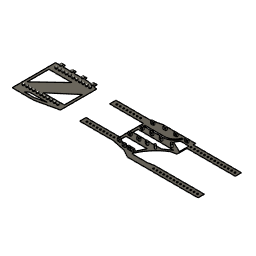
palm&backhand v9 (Autodesk Fusion 360 design; units mm, degrees)
Autodesk Fusion 360 part; units mm, degrees
(part 1 of 4)
sketch "Sketch1" plane through (0, 0, 0) normal (0, 0, 1) x (1, 0, 0)
  line L0 (90, 80) -> (90, -10)
  line L1 (45, 80) -> (45, -10) construction
  line L2 (45, -10) -> (0, 0)
  line L3 (45, -10) -> (90, -10)
  line L4 (22.5, 80) -> (90, 80)
  line L5 (22.5, 80) -> (0, 75)
  line L6 (0, 0) -> (0, 75)
  line L7 (90, 80) -> (90, 40) construction
  arc A0 (90, 40) -> (45, -10) centre (128.4491, -39.8542) ccw
  arc A1 (87.8309, 44.505) -> (40.2922, -8.3158) centre (128.4491, -39.8542) ccw
  line L8 (87.8309, 44.505) -> (87.8309, 38.9188)
  line L9 (87.8309, 44.505) -> (90, 44.58)
  line L10 (40.6089, -7.444) -> (45.6219, -8.3158)
  line L11 (40.2922, -8.3158) -> (40.0807, -8.9068)
  line L12 (0, 0) -> (-30, 0)
  line L13 (-30, 0) -> (-30, 75)
  line L14 (-30, 75) -> (0, 75)
  line L15 (-30, 5) -> (0, 5)
  line L16 (-30, 70) -> (0, 70)
  line L17 (-75, -10) -> (-30, 0)
  line L18 (-117.8309, 44.505) -> (-117.8309, 38.9188)
  line L19 (-70.6089, -7.444) -> (-75.6219, -8.3158)
  line L20 (-120, 80) -> (-120, 40) construction
  line L21 (-120, 80) -> (-120, -10)
  line L22 (-75, 80) -> (-75, -10) construction
  arc A2 (-120, 40) -> (-75, -10) centre (-158.4491, -39.8542) cw
  line L23 (-52.5, 80) -> (-120, 80)
  arc A3 (-117.8309, 44.505) -> (-70.2922, -8.3158) centre (-158.4491, -39.8542) cw
  line L24 (-70.2922, -8.3158) -> (-70.0807, -8.9068)
  line L25 (-117.8309, 44.505) -> (-120, 44.58)
  line L26 (-75, -10) -> (-120, -10)
  line L27 (-52.5, 80) -> (-30, 75)
  line L28 (90, 80) -> (90, 75)
  line L29 (90, 44.58) -> (89.8272, 49.577)
  line L30 (90, 75) -> (190, 75)
  line L31 (75.7574, -10) -> (181.8234, -116.066)
  line L32 (181.8234, -116.066) -> (195.9655, -101.9239)
  line L33 (195.9655, -101.9239) -> (89.8995, 4.1421)
  line L34 (89.8995, 4.1421) -> (75.7574, -10)
  circle A4 centre (187.1267, -107.2272) radius 2.5 construction
  circle A5 centre (181.8234, -101.9239) radius 5
  circle A6 centre (174.7523, -94.8528) radius 5 construction
  circle A7 centre (167.6812, -87.7817) radius 5
  circle A8 centre (160.6102, -80.7107) radius 5 construction
  circle A9 centre (153.5391, -73.6396) radius 5
  circle A10 centre (146.468, -66.5685) radius 5 construction
  circle A11 centre (139.397, -59.4975) radius 5
  circle A12 centre (132.3259, -52.4264) radius 5 construction
  line L35 (188.8944, -108.9949) -> (82.8284, -2.9289) construction
  circle A13 centre (125.2548, -45.3553) radius 5
  circle A14 centre (118.1838, -38.2843) radius 5 construction
  circle A15 centre (111.1127, -31.2132) radius 5
  line L36 (190, 62.2885) -> (90, 62.2885)
  line L37 (90, 75) -> (90, 62.2885)
  line L38 (190, 62.2885) -> (190, 75)
  line L39 (190, 68.6442) -> (90, 68.6442) construction
  circle A16 centre (187.5, 68.6442) radius 2.5 construction
  circle A17 centre (180, 68.6442) radius 5
  circle A18 centre (170, 68.6442) radius 5 construction
  circle A19 centre (160, 68.6442) radius 5
  circle A20 centre (150, 68.6442) radius 5 construction
  circle A21 centre (140, 68.6442) radius 5
  circle A22 centre (130, 68.6442) radius 5 construction
  circle A23 centre (120, 68.6442) radius 5
  circle A24 centre (111.1127, -31.2132) radius 4.5
  circle A25 centre (125.2548, -45.3553) radius 4.5
  circle A26 centre (139.397, -59.4975) radius 4.5
  circle A27 centre (153.5391, -73.6396) radius 4.5
  circle A28 centre (167.6812, -87.7817) radius 4.5
  circle A29 centre (181.8234, -101.9239) radius 4.5
  circle A30 centre (104.0416, -24.1421) radius 5 construction
  circle A31 centre (96.9706, -17.0711) radius 5 construction
  circle A32 centre (96.9706, -17.0711) radius 4.5
  dimension "d3" = 90
  dimension "d4" = 90
  dimension "d7" = 40
  dimension "d8" = 5
  dimension "d9" = 30
  dimension "d13" = 90
  dimension "d14" = 90
  dimension "d15" = 40
  dimension "d16" = 5
  dimension "d17" = 5
  dimension "d18" = 100
  dimension "d20" = 150
  dimension "d22" = 5
  dimension "d23" = 10
  dimension "d24" = 10
  dimension "d25" = 10
  dimension "d26" = 10
  dimension "d27" = 10
  dimension "d28" = 10
  dimension "d29" = 10
  dimension "d30" = 10
  dimension "d31" = 10
  dimension "d32" = 10
  dimension "d33" = 10
  dimension "d34" = 5
  dimension "d35" = 10
  dimension "d36" = 10
  dimension "d37" = 10
  dimension "d38" = 10
  dimension "d39" = 10
  dimension "d40" = 10
  dimension "d41" = 10
  dimension "d465" = 9
  dimension "d466" = 9
  dimension "d467" = 9
  dimension "d468" = 9
  dimension "d469" = 9
  dimension "d470" = 9
  dimension "d539" = 10
  dimension "d540" = 10
  dimension "d541" = 9
  constraint coincident L2.end L6.start
  constraint perpendicular L0 L4
  constraint vertical L6
  constraint perpendicular L4 L7
  constraint coincident A0 L8.end
  constraint vertical L8
  constraint coincident L0 L9.end
  constraint coincident A1 L10.start
  constraint coincident A0 L10.end
  constraint coincident L2 L11.end
  constraint tangent A1 L11
  constraint perpendicular L6 L12
  constraint perpendicular L12 L13
  constraint perpendicular L6 L14
  constraint coincident L13 L15.start
  constraint coincident L6 L15.end
  constraint perpendicular L6 L15
  constraint coincident L13 L16.start
  constraint coincident L6 L16.end
  constraint perpendicular L6 L16
  constraint perpendicular L21 L23
  constraint perpendicular L20 L23
  constraint coincident L18.end A2
  constraint coincident L25.end L21
  constraint coincident L19.start A3
  constraint coincident L19.end A2
  constraint coincident L24.end L17
  constraint tangent A3 L24
  constraint concentric A2 A3
  constraint perpendicular L4 L28
  constraint perpendicular L9 L29
  constraint horizontal L30
  constraint midpoint L32 L35.start
  constraint midpoint L34 L35.end
  constraint perpendicular L0 L36
  constraint perpendicular L36 L37
  constraint perpendicular L30 L38
  constraint midpoint L38 L39.start
  constraint midpoint L37 L39.end
  constraint perpendicular L7 L39
  constraint coincident L39.start A16
  constraint concentric A15 A24
  constraint concentric A13 A25
  constraint concentric A11 A26
  constraint concentric A9 A27
  constraint concentric A7 A28
  constraint concentric A5 A29
  constraint concentric A31 A32
  measures "d3" distance of L0.start L0.end
  measures "d4" distance of L1.start L1.end
  measures "d7" distance of L0.start L7.end
  measures "d9" distance of L2.end L12.end
  measures "d13" distance of L21.end L20.start
  measures "d14" distance of L17.start L22.start
  measures "d15" distance of L20.end L20.start
  measures "d16" distance of L0.start L28.end
  measures "d17" distance of L9.end L29.end
  measures "d18" distance of L28.end L30.end
  measures "d20" distance of L31.start L31.end
  measures "d22" diameter of A4
  measures "d23" diameter of A5
  measures "d24" diameter of A6
  measures "d25" diameter of A7
  measures "d26" diameter of A8
  measures "d27" diameter of A9
  measures "d28" diameter of A10
  measures "d29" diameter of A11
  measures "d30" diameter of A12
  measures "d31" diameter of A13
  measures "d32" diameter of A14
  measures "d33" diameter of A15
  measures "d34" diameter of A16
  measures "d35" diameter of A17
  measures "d36" diameter of A18
  measures "d37" diameter of A19
  measures "d38" diameter of A20
  measures "d39" diameter of A21
  measures "d40" diameter of A22
  measures "d41" diameter of A23
  measures "d465" diameter of A24
  measures "d466" diameter of A25
  measures "d467" diameter of A26
  measures "d468" diameter of A27
  measures "d469" diameter of A28
  measures "d470" diameter of A29
  measures "d539" diameter of A30
  measures "d540" diameter of A31
  measures "d541" diameter of A32
extrude "Extrude1" add sketch "Sketch1" along normal blind 0.5 contours L0 L2 L4 L5 L6 A1 L9 L11 L28 L37 | L0 L30 L36 L37 L38 | L6 L13 L14 L16 | L0 A0 L8 L9 | L13 L17 L21 L23 A3 L24 L25 L27 | L0 L3 A0 L33 L34 | L6 L12 L13 L15 | L0 L3 L31 L32 L33 | L0 L3 L33 L34 | L2 A0 A1 L10 L11 | L18 L21 A2 L25 | L17 L19 A2 A3 L24 | L21 A2 L26 | L18 L19 A2 A3 | A32 makes body 1
sketch "Sketch2" plane through (0, 0, 0.5) normal (0, 0, 1) x (-1, 0, 0)
  line L0 (0, -5) -> (30, -5)
  line L1 (30, -5) -> (30, -70)
  line L2 (30, -70) -> (0, -70)
  line L3 (0, -70) -> (0, -5)
  circle A0 centre (-167.6812, 87.7817) radius 5
  circle A1 centre (-120, -68.6442) radius 5
  circle A2 centre (-140, -68.6442) radius 5
  circle A3 centre (-153.5391, 73.6396) radius 5
  arc A4 (-87.8309, -44.505) -> (-40.6089, 7.444) centre (-128.4491, 39.8542) ccw
  line L4 (-87.8309, -44.505) -> (-87.8309, -38.9188)
  arc A5 (-87.8309, -38.9188) -> (-45.6219, 8.3158) centre (-128.4491, 39.8542) ccw
  line L5 (-45.6219, 8.3158) -> (-40.6089, 7.444)
  circle A6 centre (-181.8234, 101.9239) radius 5
  circle A7 centre (-160, -68.6442) radius 5
  circle A8 centre (-180, -68.6442) radius 5
  circle A9 centre (-139.397, 59.4975) radius 5
  circle A10 centre (-125.2548, 45.3553) radius 5
  circle A11 centre (-111.1127, 31.2132) radius 5
  line L6 (-90, -62.2885) -> (-190, -62.2885)
  line L7 (-190, -62.2885) -> (-190, -75)
  line L8 (-190, -75) -> (-90, -75)
  line L9 (-90, -75) -> (-90, -80)
  line L10 (-90, -80) -> (-22.5, -80)
  line L11 (-22.5, -80) -> (0, -75)
  line L12 (0, -75) -> (30, -75)
  line L13 (30, -75) -> (52.5, -80)
  line L14 (52.5, -80) -> (120, -80)
  line L15 (120, -80) -> (120, 10)
  line L16 (120, 10) -> (75, 10)
  line L17 (75, 10) -> (30, 0)
  line L18 (30, 0) -> (0, 0)
  line L19 (0, 0) -> (-45, 10)
  line L20 (-45, 10) -> (-75.7574, 10)
  line L21 (-75.7574, 10) -> (-181.8234, 116.066)
  line L22 (-181.8234, 116.066) -> (-195.9655, 101.9239)
  line L23 (-195.9655, 101.9239) -> (-90, -4.0416)
  line L24 (-90, -4.0416) -> (-90, -62.2885)
  line L25 (-87.8309, -38.9188) -> (-87.8309, 22.0735) construction
  line L26 (-45.6219, 8.3158) -> (-102.3574, 8.3158) construction
  line L27 (-87.8309, -38.9188) -> (-90, -38.9188) construction
  line L28 (-90, -38.9188) -> (-90, -4.0416) construction
  line L29 (-51.4544, -4.0416) -> (-90, -4.0416) construction
  line L30 (-75.7574, 10) -> (-75.7574, -31.4101) construction
  line L31 (-87.8309, -29.9541) -> (-85.8309, -29.9541)
  line L32 (-85.8309, -29.9541) -> (-85.8309, -27.9541)
  line L33 (-85.8309, -27.9541) -> (-87.8309, -27.9541)
  line L34 (-87.8309, -27.9541) -> (-87.8309, -29.9541)
  line L35 (-87.8309, -21.8881) -> (-85.8309, -21.8881)
  line L36 (-85.8309, -21.8881) -> (-85.8309, -19.8881)
  line L37 (-85.8309, -19.8881) -> (-87.8309, -19.8881)
  line L38 (-87.8309, -19.8881) -> (-87.8309, -21.8881)
  line L39 (-71.5164, -21.5952) -> (-72.9306, -23.0095)
  line L40 (-72.9306, -23.0095) -> (-74.3448, -21.5952)
  line L41 (-74.3448, -21.5952) -> (-72.9306, -20.181)
  line L42 (-72.9306, -20.181) -> (-71.5164, -21.5952)
  line L43 (-75.5164, -17.5952) -> (-76.9306, -19.0095)
  line L44 (-76.9306, -19.0095) -> (-78.3448, -17.5952)
  line L45 (-78.3448, -17.5952) -> (-76.9306, -16.181)
  line L46 (-76.9306, -16.181) -> (-75.5164, -17.5952)
  line L47 (-68.8009, -7.396) -> (-69.6461, -9.2087)
  line L48 (-69.6461, -9.2087) -> (-71.4587, -8.3634)
  line L49 (-71.4587, -8.3634) -> (-70.6135, -6.5508)
  line L50 (-70.6135, -6.5508) -> (-68.8009, -7.396)
  line L51 (-63.674, -9.7867) -> (-64.5193, -11.5994)
  line L52 (-64.5193, -11.5994) -> (-66.3319, -10.7541)
  line L53 (-65.4866, -8.9415) -> (-63.674, -9.7867)
  line L54 (-66.3319, -10.7541) -> (-65.4866, -8.9415)
  line L55 (-65.8203, 7.9003) -> (-65.8203, 5.9003)
  line L56 (-65.8203, 5.9003) -> (-67.8203, 5.9003)
  line L57 (-67.8203, 5.9003) -> (-67.8203, 7.9003)
  line L58 (-67.8203, 7.9003) -> (-65.8203, 7.9003)
  line L59 (-60.1634, 7.9003) -> (-60.1634, 5.9003)
  line L60 (-60.1634, 5.9003) -> (-62.1634, 5.9003)
  line L61 (-62.1634, 7.9003) -> (-60.1634, 7.9003)
  line L62 (-62.1634, 5.9003) -> (-62.1634, 7.9003)
  line L63 (-22.5, -80) -> (-22.5, 5)
  line L64 (0, -75) -> (0, 0)
  line L65 (0, -70) -> (-22.5, -70)
  line L66 (-14.25, -71.5) -> (-8.25, -71.5)
  line L67 (-8.25, -71.5) -> (-8.25, -68.5)
  line L68 (-8.25, -68.5) -> (-14.25, -68.5)
  line L69 (-14.25, -68.5) -> (-14.25, -71.5)
  line L70 (-14.25, -71.5) -> (-8.25, -68.5) construction
  line L71 (-8.25, -71.5) -> (-14.25, -68.5) construction
  line L72 (-22.5, -80) -> (-45, -80)
  line L73 (-45, -80) -> (-67.5, -80)
  line L74 (-45, -80) -> (-45, 10) construction
  line L75 (-67.5, -80) -> (-67.5, 10) construction
  line L76 (-33.75, -80) -> (-33.75, 7.5) construction
  line L77 (-56.25, -80) -> (-56.25, 10) construction
  line L78 (-67.5, -80) -> (-90, -80) construction
  line L79 (-78.75, -80) -> (-78.75, 12.9926) construction
  line L80 (-36.75, -74.5367) -> (-30.75, -74.5367)
  line L81 (-30.75, -74.5367) -> (-30.75, -71.5367)
  line L82 (-30.75, -71.5367) -> (-36.75, -71.5367)
  line L83 (-36.75, -71.5367) -> (-36.75, -74.5367)
  line L84 (-36.75, -74.5367) -> (-30.75, -71.5367) construction
  line L85 (-30.75, -74.5367) -> (-36.75, -71.5367) construction
  line L86 (-33.75, -73.0367) -> (-78.75, -73.0367) construction
  line L87 (-59.25, -74.5367) -> (-53.25, -74.5367)
  line L88 (-53.25, -74.5367) -> (-53.25, -71.5367)
  line L89 (-53.25, -71.5367) -> (-59.25, -71.5367)
  line L90 (-59.25, -71.5367) -> (-59.25, -74.5367)
  line L91 (-59.25, -74.5367) -> (-53.25, -71.5367) construction
  line L92 (-53.25, -74.5367) -> (-59.25, -71.5367) construction
  line L93 (-81.75, -74.5367) -> (-75.75, -74.5367)
  line L94 (-75.75, -74.5367) -> (-75.75, -71.5367)
  line L95 (-75.75, -71.5367) -> (-81.75, -71.5367)
  line L96 (-81.75, -71.5367) -> (-81.75, -74.5367)
  line L97 (-81.75, -74.5367) -> (-75.75, -71.5367) construction
  line L98 (-75.75, -74.5367) -> (-81.75, -71.5367) construction
  line L99 (0, -70) -> (0, -50) construction
  line L100 (0, -50) -> (-90, -50) construction
  line L101 (0, -50) -> (0, -30) construction
  line L102 (0, -30) -> (-90, -30.3753) construction
  line L103 (0, -30) -> (0, -10) construction
  line L104 (0, -10) -> (-90, -10.0044) construction
  line L105 (-12.5179, -50.929) -> (-6.6181, -52.0209)
  line L106 (-6.6181, -52.0209) -> (-6.0721, -49.071)
  line L107 (-6.0721, -49.071) -> (-11.9719, -47.9791)
  line L108 (-11.9719, -47.9791) -> (-12.5179, -50.929)
  line L109 (-12.5179, -50.929) -> (-6.0721, -49.071) construction
  line L110 (-6.6181, -52.0209) -> (-11.9719, -47.9791) construction
  line L111 (-26.1784, -49.0328) -> (-32.0908, -48.011)
  line L112 (-32.0908, -48.011) -> (-32.6017, -50.9672)
  line L113 (-32.6017, -50.9672) -> (-26.6893, -51.989)
  line L114 (-26.6893, -51.989) -> (-26.1784, -49.0328)
  line L115 (-26.1784, -49.0328) -> (-32.6017, -50.9672) construction
  line L116 (-32.0908, -48.011) -> (-26.6893, -51.989) construction
  line L117 (-51.8014, -50.3661) -> (-46.174, -52.4476)
  line L118 (-46.174, -52.4476) -> (-45.1333, -49.6339)
  line L119 (-45.1333, -49.6339) -> (-50.7607, -47.5524)
  line L120 (-50.7607, -47.5524) -> (-51.8014, -50.3661)
  line L121 (-51.8014, -50.3661) -> (-45.1333, -49.6339) construction
  line L122 (-46.174, -52.4476) -> (-50.7607, -47.5524) construction
  line L123 (-73.9232, -49.4996) -> (-69.0348, -52.9787)
  line L124 (-69.0348, -52.9787) -> (-67.271, -50.5004)
  line L125 (-67.271, -50.5004) -> (-72.1594, -47.0213)
  line L126 (-72.1594, -47.0213) -> (-73.9232, -49.4996)
  line L127 (-73.9232, -49.4996) -> (-67.271, -50.5004) construction
  line L128 (-69.0348, -52.9787) -> (-72.1594, -47.0213) construction
  line L129 (-59.9232, -29.4996) -> (-55.0348, -32.9787)
  line L130 (-55.0348, -32.9787) -> (-53.271, -30.5004)
  line L131 (-53.271, -30.5004) -> (-58.1594, -27.0213)
  line L132 (-58.1594, -27.0213) -> (-59.9232, -29.4996)
  line L133 (-44.8014, -28.3661) -> (-39.174, -30.4476)
  line L134 (-39.174, -30.4476) -> (-38.1333, -27.6339)
  line L135 (-38.1333, -27.6339) -> (-43.7607, -25.5524)
  line L136 (-43.7607, -25.5524) -> (-44.8014, -28.3661)
  line L137 (-28.6017, -27.9672) -> (-22.6893, -28.989)
  line L138 (-22.6893, -28.989) -> (-22.1784, -26.0328)
  line L139 (-22.1784, -26.0328) -> (-28.0908, -25.011)
  line L140 (-28.0908, -25.011) -> (-28.6017, -27.9672)
  line L141 (-10.5982, -28.1022) -> (-4.5984, -28.1531)
  line L142 (-4.5984, -28.1531) -> (-4.573, -25.1532)
  line L143 (-4.573, -25.1532) -> (-10.5728, -25.1023)
  line L144 (-10.5728, -25.1023) -> (-10.5982, -28.1022)
  line L145 (-10.5982, -6.1022) -> (-4.5984, -6.1531)
  line L146 (-4.5984, -6.1531) -> (-4.573, -3.1532)
  line L147 (-4.573, -3.1532) -> (-10.5728, -3.1023)
  line L148 (-10.5728, -3.1023) -> (-10.5982, -6.1022)
  line L149 (-24.6759, -2.141) -> (-18.6759, -2.1206)
  line L150 (-18.6759, -2.1206) -> (-18.6861, 0.8794)
  line L151 (-18.6861, 0.8794) -> (-24.686, 0.859)
  line L152 (-24.686, 0.859) -> (-24.6759, -2.141)
  line L153 (-35.048, -2.0492) -> (-29.0481, -2.0804)
  line L154 (-29.0481, -2.0804) -> (-29.0325, 0.9195)
  line L155 (-29.0325, 0.9195) -> (-35.0324, 0.9507)
  line L156 (-35.0324, 0.9507) -> (-35.048, -2.0492)
  line L157 (-42.2023, -1.9219) -> (-36.2025, -1.9678)
  line L158 (-36.2025, -1.9678) -> (-36.1792, 1.0739)
  line L159 (-36.1792, 1.0739) -> (-42.179, 1.1199)
  line L160 (-42.179, 1.1199) -> (-42.2023, -1.9219)
  line L161 (0, -60) -> (-22.5, -60)
  line L162 (-22.5, -60) -> (-45, -60)
  arc A12 (-45, -60) -> (-67.5, -80) centre (-45, -82.6562) ccw
  line L163 (0, -57) -> (-22.5, -57)
  line L164 (-22.5, -57) -> (-45, -57)
  arc A13 (-45, -57) -> (-70.4793, -79.6483) centre (-45, -82.6562) ccw
  line L165 (-70.4793, -79.6483) -> (-70.4683, -80)
  line L166 (0, -58.3775) -> (-5, -58.3775)
  line L167 (-5, -60) -> (-5, -57)
  line L168 (-68.9513, -80) -> (-68.9513, -75)
  line L169 (-69.4872, -75) -> (-66.3234, -75)
  point P0 (-11.25, -70)
  point P1 (-33.75, -73.0367)
  point P2 (-56.25, -73.0367)
  point P3 (-78.75, -73.0367)
  point P4 (-9.295, -50)
  point P5 (-29.39, -50)
  point P6 (-48.4674, -50)
  point P7 (-70.5971, -50)
  dimension "d44" = 2
  dimension "d45" = 2
  dimension "d46" = 2
  dimension "d47" = 2
  dimension "d48" = 2
  dimension "d49" = 2
  dimension "d50" = 2
  dimension "d51" = 2
  dimension "d52" = 2
  dimension "d53" = 2
  dimension "d54" = 2
  dimension "d55" = 2
  dimension "d56" = 2
  dimension "d57" = 2
  dimension "d58" = 2
  dimension "d59" = 2
  dimension "d60" = 6
  dimension "d61" = 3
  dimension "d62" = 22.5
  dimension "d63" = 22.5
  dimension "d64" = 6
  dimension "d65" = 3
  dimension "d66" = 6
  dimension "d67" = 3
  dimension "d68" = 6
  dimension "d69" = 3
  dimension "d70" = 20
  dimension "d71" = 20
  dimension "d72" = 20
  dimension "d73" = 6
  dimension "d74" = 3
  dimension "d75" = 6
  dimension "d76" = 3
  dimension "d77" = 6
  dimension "d78" = 3
  dimension "d79" = 6
  dimension "d80" = 6
  dimension "d81" = 6
  dimension "d82" = 3
  dimension "d83" = 6
  dimension "d84" = 3
  dimension "d85" = 6
  dimension "d86" = 3
  dimension "d87" = 6
  dimension "d88" = 3
  dimension "d89" = 6
  dimension "d90" = 3
  dimension "d91" = 6
  dimension "d92" = 3
  dimension "d93" = 6
  dimension "d94" = 3
  dimension "d95" = 5
  dimension "d96" = 5
  constraint coincident L4.end A5.start
  constraint coincident L21 L25.end
  constraint parallel L4 L25
  constraint coincident A5.end L5.start
  constraint coincident L23 L26.end
  constraint perpendicular L25 L26
  constraint coincident L24 L27.end
  constraint perpendicular L24 L27
  constraint coincident L23.end L24.start
  constraint coincident A5 L29.start
  constraint perpendicular L28 L29
  constraint coincident L20.end L21.start
  constraint coincident A5 L30.end
  constraint perpendicular L26 L30
  constraint horizontal L31
  constraint vertical L32
  constraint horizontal L33
  constraint vertical L34
  constraint coincident L25 L31.start
  constraint horizontal L35
  constraint vertical L36
  constraint horizontal L37
  constraint vertical L38
  constraint coincident L25 L35.start
  constraint coincident L10.end L11.start
  constraint midpoint L19 L63.end
  constraint coincident L11.end L12.start
  constraint coincident L18.end L19.start
  constraint coincident L2.end L3.start
  constraint coincident L63 L65.end
  constraint perpendicular L63 L65
  constraint horizontal L66
  constraint perpendicular L66 L67
  constraint parallel L66 L68
  constraint parallel L67 L69
  constraint coincident L70 P0
  constraint coincident L71 P0
  constraint midpoint L65 P0
  constraint coincident L10 L72.end
  constraint coincident L10 L73.end
  constraint coincident L19.end L20.start
  constraint coincident L20 L75.end
  constraint perpendicular L20 L75
  constraint midpoint L72 L76.start
  constraint coincident L19 L76.end
  constraint perpendicular L10 L76
  constraint midpoint L10 L77.start
  constraint coincident L20 L77.end
  constraint perpendicular L20 L77
  constraint coincident L9.end L10.start
  constraint midpoint L78 L79.start
  constraint coincident L21 L79.end
  constraint perpendicular L20 L79
  constraint horizontal L80
  constraint perpendicular L80 L81
  constraint parallel L80 L82
  constraint parallel L81 L83
  constraint coincident L84 P1
  constraint coincident L85 P1
  constraint coincident L76 P1
  constraint coincident P1 L86.start
  constraint coincident L79 P3
  constraint perpendicular L79 L86
  constraint horizontal L87
  constraint perpendicular L87 L88
  constraint parallel L87 L89
  constraint parallel L88 L90
  constraint coincident L91 P2
  constraint coincident L92 P2
  constraint midpoint L86 P2
  constraint horizontal L93
  constraint perpendicular L93 L94
  constraint parallel L93 L95
  constraint parallel L94 L96
  constraint coincident L97 P3
  constraint coincident L98 P3
  constraint coincident P3 L86.end
  constraint coincident L64 L99.end
  constraint coincident L24 L100.end
  constraint perpendicular L24 L100
  constraint coincident L64 L101.end
  constraint coincident L28 L102.end
  constraint coincident L64 L103.end
  constraint coincident L28 L104.end
  constraint perpendicular L105 L106
  constraint parallel L105 L107
  constraint parallel L106 L108
  constraint coincident L109 P4
  constraint coincident L110 P4
  constraint coincident L100 P4
  constraint perpendicular L111 L112
  constraint parallel L111 L113
  constraint parallel L112 L114
  constraint coincident L115 P5
  constraint coincident L116 P5
  constraint coincident L100 P5
  constraint perpendicular L117 L118
  constraint parallel L117 L119
  constraint parallel L118 L120
  constraint coincident L121 P6
  constraint coincident L122 P6
  constraint coincident L100 P6
  constraint perpendicular L123 L124
  constraint parallel L123 L125
  constraint parallel L124 L126
  constraint coincident L127 P7
  constraint coincident L128 P7
  constraint coincident L100 P7
  constraint perpendicular L129 L130
  constraint parallel L129 L131
  constraint parallel L130 L132
  constraint perpendicular L133 L134
  constraint parallel L133 L135
  constraint parallel L134 L136
  constraint perpendicular L139 L140
  constraint parallel L137 L139
  constraint parallel L138 L140
  constraint perpendicular L141 L142
  constraint parallel L141 L143
  constraint parallel L142 L144
  constraint perpendicular L145 L146
  constraint parallel L145 L147
  constraint parallel L146 L148
  constraint perpendicular L151 L152
  constraint parallel L149 L151
  constraint parallel L150 L152
  constraint perpendicular L153 L154
  constraint parallel L153 L155
  constraint parallel L154 L156
  constraint perpendicular L157 L158
  constraint parallel L157 L159
  constraint parallel L158 L160
  constraint midpoint L99 L161.start
  constraint coincident L63 L161.end
  constraint perpendicular L63 L161
  constraint coincident L74 L162.end
  constraint perpendicular L74 L162
  constraint tangent L162 A12
  constraint coincident L78 L165.end
  constraint coincident L64 L166.start
  constraint perpendicular L64 L166
  constraint coincident L161 L167.start
  constraint coincident L163 L167.end
  constraint perpendicular L163 L167
  constraint coincident L78 L168.start
  constraint perpendicular L78 L168
  constraint coincident A13 L169.start
  constraint coincident A12 L169.end
  constraint perpendicular L75 L169
  measures "d44" distance of L31.start L31.end
  measures "d45" distance of L31.start L33.end
  measures "d46" distance of L35.start L35.end
  measures "d47" distance of L35.start L37.end
  measures "d48" distance of L39.start L39.end
  measures "d49" distance of L39.start L41.end
  measures "d50" distance of L43.start L43.end
  measures "d51" distance of L43.start L45.end
  measures "d52" distance of L51.start L51.end
  measures "d53" distance of L51.start L53.start
  measures "d54" distance of L47.start L47.end
  measures "d55" distance of L47.start L49.end
  measures "d56" distance of L59.end L59.start
  measures "d57" distance of L59.start L61.start
  measures "d58" distance of L55.start L55.end
  measures "d59" distance of L55.start L57.end
  measures "d60" distance of L67.end L68.end
  measures "d61" distance of L66.end L67.end
  measures "d62" distance of L10.end L72.end
  measures "d63" distance of L72.end L73.end
  measures "d64" distance of L81.end L82.end
  measures "d65" distance of L80.end L81.end
  measures "d66" distance of L88.end L89.end
  measures "d67" distance of L87.end L88.end
  measures "d68" distance of L94.end L95.end
  measures "d69" distance of L93.end L94.end
  measures "d70" distance of L2.end L99.end
  measures "d71" distance of L99.end L101.end
  measures "d72" distance of L101.end L103.end
  measures "d73" distance of L106.end L107.end
  measures "d74" distance of L105.end L106.end
  measures "d75" distance of L112.end L113.end
  measures "d76" distance of L111.end L112.end
  measures "d77" distance of L118.end L119.end
  measures "d78" distance of L117.end L118.end
  measures "d79" distance of L124.end L125.end
  measures "d80" distance of L130.end L131.end
  measures "d81" distance of L134.end L135.end
  measures "d82" distance of L133.end L134.end
  measures "d83" distance of L137.start L137.end
  measures "d84" distance of L137.start L139.end
  measures "d85" distance of L142.end L143.end
  measures "d86" distance of L142.end L141.end
  measures "d87" distance of L146.end L147.end
  measures "d88" distance of L145.end L146.end
  measures "d89" distance of L149.start L149.end
  measures "d90" distance of L149.start L151.end
  measures "d91" distance of L154.end L155.end
  measures "d92" distance of L153.end L154.end
  measures "d93" distance of L159.end L158.end
  measures "d95" distance of L166.start L166.end
  measures "d96" distance of L168.start L168.end
extrude "Extrude2" cut sketch "Sketch2" against normal blind 15 contours L63 L161 L163 L167 | L63 L162 A12 L164 A13 L169 bodies 1
extrude "Extrude3" add sketch "Sketch2" along normal blind 1.5 contours L63 L149 L150 L151 | L63 L149 L151 L152 | L65 L66 L67 L69 | L65 L67 L68 L69 | L63 L137 L138 L139 L140 | L63 L138 L139 | L31 L32 L33 L34 | L35 L36 L37 L38 | L39 L40 L41 L42 | L43 L44 L45 L46 | L47 L48 L49 L50 | L51 L52 L53 L54 | L55 L56 L57 L58 | L59 L60 L61 L62 | L80 L81 L82 L83 | L87 L88 L89 L90 | L93 L94 L95 L96 | L105 L106 L107 L108 | L111 L112 L113 L114 | L117 L118 L119 L120 | L123 L124 L125 L126 | L129 L130 L131 L132 | L133 L134 L135 L136 | L141 L142 L143 L144 | L145 L146 L147 L148 | L153 L154 L155 L156 | L157 L158 L159 L160 bodies 1
sketch "Sketch3" plane through (0, 0, 0.5) normal (0, 0, 1) x (-1, 0, 0)
  line L0 (-14.25, -68.5) -> (-8.25, -68.5)
  line L1 (-8.25, -68.5) -> (-8.25, -71.5)
  line L2 (-8.25, -71.5) -> (-14.25, -71.5)
  line L3 (-14.25, -71.5) -> (-14.25, -68.5)
  line L4 (-72.1594, -47.0213) -> (-67.271, -50.5004)
  line L5 (-67.271, -50.5004) -> (-69.0348, -52.9787)
  line L6 (-69.0348, -52.9787) -> (-73.9232, -49.4996)
  line L7 (-73.9232, -49.4996) -> (-72.1594, -47.0213)
  line L8 (-58.1594, -27.0213) -> (-53.271, -30.5004)
  line L9 (-53.271, -30.5004) -> (-55.0348, -32.9787)
  line L10 (-55.0348, -32.9787) -> (-59.9232, -29.4996)
  line L11 (-59.9232, -29.4996) -> (-58.1594, -27.0213)
  line L12 (-10.5728, -3.1023) -> (-4.573, -3.1532)
  line L13 (-4.573, -3.1532) -> (-4.5984, -6.1531)
  line L14 (-4.5984, -6.1531) -> (-10.5982, -6.1022)
  line L15 (-10.5982, -6.1022) -> (-10.5728, -3.1023)
  line L16 (-67.8203, 7.9003) -> (-65.8203, 7.9003)
  line L17 (-65.8203, 7.9003) -> (-65.8203, 5.9003)
  line L18 (-65.8203, 5.9003) -> (-67.8203, 5.9003)
  line L19 (-67.8203, 5.9003) -> (-67.8203, 7.9003)
  line L20 (-76.9306, -16.181) -> (-75.5164, -17.5952)
  line L21 (-75.5164, -17.5952) -> (-76.9306, -19.0095)
  line L22 (-76.9306, -19.0095) -> (-78.3448, -17.5952)
  line L23 (-78.3448, -17.5952) -> (-76.9306, -16.181)
  line L24 (-87.8309, -27.9541) -> (-85.8309, -27.9541)
  line L25 (-85.8309, -27.9541) -> (-85.8309, -29.9541)
  line L26 (-85.8309, -29.9541) -> (-87.8309, -29.9541)
  line L27 (-87.8309, -29.9541) -> (-87.8309, -27.9541)
  line L28 (-66.3319, -10.7541) -> (-65.4866, -8.9415)
  line L29 (-65.4866, -8.9415) -> (-63.674, -9.7867)
  line L30 (-63.674, -9.7867) -> (-64.5193, -11.5994)
  line L31 (-64.5193, -11.5994) -> (-66.3319, -10.7541)
  line L32 (-42.179, 1.1199) -> (-36.1792, 1.0739)
  line L33 (-36.1792, 1.0739) -> (-36.2025, -1.9678)
  line L34 (-36.2025, -1.9678) -> (-42.2023, -1.9219)
  line L35 (-42.2023, -1.9219) -> (-42.179, 1.1199)
  line L36 (-10.5728, -25.1023) -> (-4.573, -25.1532)
  line L37 (-4.573, -25.1532) -> (-4.5984, -28.1531)
  line L38 (-4.5984, -28.1531) -> (-10.5982, -28.1022)
  line L39 (-10.5982, -28.1022) -> (-10.5728, -25.1023)
  line L40 (-11.9719, -47.9791) -> (-6.0721, -49.071)
  line L41 (-6.0721, -49.071) -> (-6.6181, -52.0209)
  line L42 (-6.6181, -52.0209) -> (-12.5179, -50.929)
  line L43 (-12.5179, -50.929) -> (-11.9719, -47.9791)
  line L44 (-81.75, -71.5367) -> (-75.75, -71.5367)
  line L45 (-75.75, -71.5367) -> (-75.75, -74.5367)
  line L46 (-75.75, -74.5367) -> (-81.75, -74.5367)
  line L47 (-81.75, -74.5367) -> (-81.75, -71.5367)
  line L48 (-36.75, -71.5367) -> (-30.75, -71.5367)
  line L49 (-30.75, -71.5367) -> (-30.75, -74.5367)
  line L50 (-30.75, -74.5367) -> (-36.75, -74.5367)
  line L51 (-36.75, -74.5367) -> (-36.75, -71.5367)
  line L52 (-50.7607, -47.5524) -> (-45.1333, -49.6339)
  line L53 (-45.1333, -49.6339) -> (-46.174, -52.4476)
  line L54 (-46.174, -52.4476) -> (-51.8014, -50.3661)
  line L55 (-51.8014, -50.3661) -> (-50.7607, -47.5524)
  line L56 (-43.7607, -25.5524) -> (-38.1333, -27.6339)
  line L57 (-38.1333, -27.6339) -> (-39.174, -30.4476)
  line L58 (-39.174, -30.4476) -> (-44.8014, -28.3661)
  line L59 (-44.8014, -28.3661) -> (-43.7607, -25.5524)
  line L60 (-24.686, 0.859) -> (-18.6861, 0.8794)
  line L61 (-18.6861, 0.8794) -> (-18.6759, -2.1206)
  line L62 (-18.6759, -2.1206) -> (-24.6759, -2.141)
  line L63 (-24.6759, -2.141) -> (-24.686, 0.859)
  line L64 (-62.1634, 5.9003) -> (-62.1634, 7.9003)
  line L65 (-62.1634, 7.9003) -> (-60.1634, 7.9003)
  line L66 (-60.1634, 7.9003) -> (-60.1634, 5.9003)
  line L67 (-60.1634, 5.9003) -> (-62.1634, 5.9003)
  line L68 (-72.9306, -20.181) -> (-71.5164, -21.5952)
  line L69 (-71.5164, -21.5952) -> (-72.9306, -23.0095)
  line L70 (-72.9306, -23.0095) -> (-74.3448, -21.5952)
  line L71 (-74.3448, -21.5952) -> (-72.9306, -20.181)
  line L72 (-87.8309, -19.8881) -> (-85.8309, -19.8881)
  line L73 (-85.8309, -19.8881) -> (-85.8309, -21.8881)
  line L74 (-85.8309, -21.8881) -> (-87.8309, -21.8881)
  line L75 (-87.8309, -21.8881) -> (-87.8309, -19.8881)
  line L76 (-70.6135, -6.5508) -> (-68.8009, -7.396)
  line L77 (-68.8009, -7.396) -> (-69.6461, -9.2087)
  line L78 (-69.6461, -9.2087) -> (-71.4587, -8.3634)
  line L79 (-71.4587, -8.3634) -> (-70.6135, -6.5508)
  line L80 (-35.0324, 0.9507) -> (-29.0325, 0.9195)
  line L81 (-29.0325, 0.9195) -> (-29.0481, -2.0804)
  line L82 (-29.0481, -2.0804) -> (-35.048, -2.0492)
  line L83 (-35.048, -2.0492) -> (-35.0324, 0.9507)
  line L84 (-28.0908, -25.011) -> (-22.1784, -26.0328)
  line L85 (-22.1784, -26.0328) -> (-22.6893, -28.989)
  line L86 (-22.6893, -28.989) -> (-28.6017, -27.9672)
  line L87 (-28.6017, -27.9672) -> (-28.0908, -25.011)
  line L88 (-26.6893, -51.989) -> (-32.6017, -50.9672)
  line L89 (-32.6017, -50.9672) -> (-32.0908, -48.011)
  line L90 (-32.0908, -48.011) -> (-26.1784, -49.0328)
  line L91 (-26.1784, -49.0328) -> (-26.6893, -51.989)
  line L92 (-59.25, -71.5367) -> (-53.25, -71.5367)
  line L93 (-53.25, -71.5367) -> (-53.25, -74.5367)
  line L94 (-53.25, -74.5367) -> (-59.25, -74.5367)
  line L95 (-59.25, -74.5367) -> (-59.25, -71.5367)
  line L96 (-45, -57) -> (-5, -57)
  line L97 (-5, -57) -> (-5, -60)
  line L98 (-5, -60) -> (-45, -60)
  arc A0 (-45, -60) -> (-66.3234, -75) centre (-45, -82.6562) ccw
  line L99 (-66.3234, -75) -> (-69.4872, -75)
  arc A1 (-45, -57) -> (-69.4872, -75) centre (-45, -82.6562) ccw
  line L100 (0, -5) -> (30, -5)
  line L101 (30, -5) -> (30, -70)
  line L102 (30, -70) -> (0, -70)
  line L103 (0, -70) -> (0, -5)
  circle A2 centre (-167.6812, 87.7817) radius 5
  circle A3 centre (-120, -68.6442) radius 5
  circle A4 centre (-140, -68.6442) radius 5
  circle A5 centre (-153.5391, 73.6396) radius 5
  arc A6 (-87.8309, -44.505) -> (-40.6089, 7.444) centre (-128.4491, 39.8542) ccw
  line L104 (-87.8309, -44.505) -> (-87.8309, -38.9188)
  arc A7 (-87.8309, -38.9188) -> (-45.6219, 8.3158) centre (-128.4491, 39.8542) ccw
  line L105 (-45.6219, 8.3158) -> (-40.6089, 7.444)
  circle A8 centre (-181.8234, 101.9239) radius 5
  circle A9 centre (-160, -68.6442) radius 5
  circle A10 centre (-180, -68.6442) radius 5
  circle A11 centre (-139.397, 59.4975) radius 5
  circle A12 centre (-125.2548, 45.3553) radius 5
  circle A13 centre (-111.1127, 31.2132) radius 5
  line L106 (-90, -62.2885) -> (-190, -62.2885)
  line L107 (-190, -62.2885) -> (-190, -75)
  line L108 (-190, -75) -> (-90, -75)
  line L109 (-90, -75) -> (-90, -80)
  line L110 (-90, -80) -> (-22.5, -80)
  line L111 (-22.5, -80) -> (0, -75)
  line L112 (0, -75) -> (30, -75)
  line L113 (30, -75) -> (52.5, -80)
  line L114 (52.5, -80) -> (120, -80)
  line L115 (120, -80) -> (120, 10)
  line L116 (120, 10) -> (75, 10)
  line L117 (75, 10) -> (30, 0)
  line L118 (30, 0) -> (0, 0)
  line L119 (0, 0) -> (-45, 10)
  line L120 (-45, 10) -> (-75.7574, 10)
  line L121 (-75.7574, 10) -> (-181.8234, 116.066)
  line L122 (-181.8234, 116.066) -> (-195.9655, 101.9239)
  line L123 (-195.9655, 101.9239) -> (-90, -4.0416)
  line L124 (-90, -4.0416) -> (-90, -62.2885)
  line L125 (-190, -68.6442) -> (120, -68.6442) construction
  line L126 (97.5, 10) -> (120, -12.5) construction
  line L127 (97.5, 10) -> (129.3198, 10) construction
  line L128 (120, 10) -> (108.75, -1.25) construction
  circle A14 centre (108.75, -1.25) radius 5
  line L129 (108.75, -1.25) -> (34.0909, -75.9091) construction
  line L130 (108.75, -1.25) -> (214.3339, -1.25) construction
  circle A15 centre (101.6789, -8.3211) radius 5
  circle A16 centre (94.6079, -15.3921) radius 5 construction
  circle A17 centre (87.5368, -22.4632) radius 5
  circle A18 centre (80.4657, -29.5343) radius 5 construction
  circle A19 centre (73.3947, -36.6053) radius 5
  circle A20 centre (117.5, -68.6442) radius 2.5
  circle A21 centre (110, -68.6442) radius 5
  circle A22 centre (100, -68.6442) radius 5 construction
  circle A23 centre (90, -68.6442) radius 5
  circle A24 centre (80, -68.6442) radius 5 construction
  circle A25 centre (70, -68.6442) radius 5
  line L131 (52.5, -80) -> (52.5, 5)
  line L132 (52.5, -80) -> (75, -80)
  line L133 (75, -80) -> (75, 10)
  line L134 (75, -80) -> (97.5, -80)
  line L135 (97.5, -80) -> (97.5, 10)
  line L136 (120, -80) -> (97.5, -80)
  circle A26 centre (108.75, -80) radius 2
  circle A27 centre (86.25, -80) radius 2
  circle A28 centre (63.75, -80) radius 2
  circle A29 centre (41.25, -77.5) radius 2
  line L137 (106.75, -80) -> (104.75, -80)
  line L138 (110.75, -80) -> (112.75, -80)
  line L139 (88.25, -80) -> (90.25, -80)
  line L140 (84.25, -80) -> (82.25, -80)
  line L141 (65.75, -80) -> (67.75, -80)
  line L142 (61.75, -80) -> (59.75, -80)
  line L143 (43.2024, -77.9339) -> (45.1547, -78.3677)
  line L144 (39.2976, -77.0661) -> (37.3453, -76.6323)
  line L145 (104.75, -80) -> (112.75, -80)
  line L146 (112.75, -80) -> (112.75, -85)
  line L147 (112.75, -85) -> (104.75, -85)
  line L148 (104.75, -85) -> (104.75, -80)
  line L149 (90.25, -80) -> (82.25, -80)
  line L150 (82.25, -80) -> (82.25, -85)
  line L151 (82.25, -85) -> (90.25, -85)
  line L152 (90.25, -85) -> (90.25, -80)
  line L153 (67.75, -80) -> (59.75, -80)
  line L154 (59.75, -80) -> (59.75, -85)
  line L155 (59.75, -85) -> (67.75, -85)
  line L156 (67.75, -85) -> (67.75, -80)
  line L157 (45.1547, -78.3677) -> (37.3453, -78.3677)
  line L158 (37.3453, -78.3677) -> (37.3453, -83.3677)
  line L159 (37.3453, -83.3677) -> (45.1547, -83.3677)
  line L160 (45.1547, -83.3677) -> (45.1547, -78.3677)
  line L161 (37.3453, -78.3677) -> (45.1547, -78.3677)
  line L162 (45.1547, -78.3677) -> (45.1547, -75.2596)
  line L163 (45.1547, -75.2596) -> (37.3453, -75.2596)
  line L164 (37.3453, -75.2596) -> (37.3453, -78.3677)
  dimension "d335" = 45
  dimension "d336" = 10
  dimension "d337" = 135
  dimension "d338" = 10
  dimension "d339" = 10
  dimension "d340" = 10
  dimension "d341" = 10
  dimension "d342" = 10
  dimension "d343" = 5
  dimension "d344" = 10
  dimension "d345" = 10
  dimension "d346" = 10
  dimension "d347" = 10
  dimension "d348" = 10
  dimension "d350" = 22.5
  dimension "d351" = 22.5
  dimension "d353" = 4
  dimension "d354" = 4
  dimension "d355" = 4
  dimension "d356" = 4
  dimension "d357" = 2
  dimension "d358" = 2
  dimension "d359" = 2
  dimension "d360" = 2
  dimension "d361" = 2
  dimension "d362" = 2
  dimension "d363" = 2
  dimension "d364" = 2
  dimension "d365" = 5
  dimension "d366" = 5
  dimension "d367" = 5
  dimension "d368" = 5
  constraint midpoint L107 L125.start
  constraint coincident L115 L125.end
  constraint perpendicular L115 L125
  constraint horizontal L127
  constraint midpoint L116 L126.start
  constraint coincident L115 L126.end
  constraint coincident L115.end L116.start
  constraint midpoint L126 L128.end
  constraint coincident L128.end A14.centre
  constraint horizontal L130
  constraint coincident L113 L129.end
  constraint coincident L125.end A20
  constraint coincident L113.end L114.start
  constraint midpoint L117 L131.end
  constraint coincident L114 L132.end
  constraint coincident L116.end L117.start
  constraint coincident L114 L134.end
  constraint coincident L114.end L115.start
  constraint midpoint L136 A26.centre
  constraint midpoint L134 A27.centre
  constraint midpoint L132 A28.centre
  constraint midpoint L113 A29.centre
  constraint coincident A26 L137.start
  constraint coincident L114 L137.start
  constraint coincident L114 L137.end
  constraint coincident A26 L138.start
  constraint coincident L136 L138.start
  constraint parallel L136 L138
  constraint coincident A27 L139.start
  constraint coincident L134 L139.start
  constraint coincident L114 L139.end
  constraint coincident A27 L140.start
  constraint coincident L134 L140.start
  constraint coincident L134 L140.end
  constraint coincident A28 L141.start
  constraint coincident L132 L141.start
  constraint coincident L132 L141.end
  constraint coincident A28 L142.start
  constraint coincident L132 L142.start
  constraint coincident L132 L142.end
  constraint coincident A29 L143.start
  constraint coincident L113 L143.start
  constraint coincident L113 L143.end
  constraint coincident A29 L144.start
  constraint coincident L113 L144.start
  constraint coincident L113 L144.end
  constraint horizontal L145
  constraint vertical L146
  constraint horizontal L147
  constraint vertical L148
  constraint horizontal L149
  constraint vertical L150
  constraint horizontal L151
  constraint vertical L152
  constraint horizontal L153
  constraint vertical L154
  constraint horizontal L155
  constraint vertical L156
  constraint horizontal L157
  constraint vertical L158
  constraint horizontal L159
  constraint vertical L160
  constraint horizontal L161
  constraint vertical L162
  constraint horizontal L163
  constraint vertical L164
  measures "d335" angle of L126 L127
  measures "d336" diameter of A14
  measures "d337" angle of L129 L130
  measures "d338" diameter of A15
  measures "d339" diameter of A16
  measures "d340" diameter of A17
  measures "d341" diameter of A18
  measures "d342" diameter of A19
  measures "d343" diameter of A20
  measures "d344" diameter of A21
  measures "d345" diameter of A22
  measures "d346" diameter of A23
  measures "d347" diameter of A24
  measures "d348" diameter of A25
  measures "d350" distance of L113.end L132.end
  measures "d351" distance of L132.end L134.end
  measures "d353" diameter of A26
  measures "d354" diameter of A27
  measures "d355" diameter of A28
  measures "d356" diameter of A29
  measures "d357" distance of L137.start L137.end
  measures "d358" distance of L138.start L138.end
  measures "d359" distance of L139.start L139.end
  measures "d360" distance of L140.start L140.end
  measures "d361" distance of L141.start L141.end
  measures "d362" distance of L142.start L142.end
  measures "d363" distance of L143.start L143.end
  measures "d364" distance of L144.start L144.end
  measures "d365" distance of L137.end L147.end
  measures "d366" distance of L139.end L151.end
  measures "d367" distance of L141.end L155.end
  measures "d368" distance of L143.end L159.end
extrude "Extrude4" add sketch "Sketch3" against normal blind 0.5 contours L113 A29 L144 L157 L161 L164 | L113 A29 L157 L161 | A29 L157 L158 L159 L160 L161 | L113 A29 L143 L157 L161 | A29 L157 L161 | L114 L132 A28 L141 L142 L153 L154 L155 L156 | L114 L132 A28 L153 | L114 L136 A26 L137 L138 L145 L146 L147 L148 | L114 L134 A27 L139 L140 L149 L150 L151 L152 | L114 L136 A26 L145 | L114 L134 A27 L149 picked at (64.3362, -81.074) picked at (108.1992, -80.5743) picked at (86.6657, -80.7199) bodies 1
extrude "Extrude5" add sketch "Sketch3" along normal blind 1.4 contours A25 | A21 | A19 L133 | A19 L133 | A15 L135 | A15 L135 | A17 | A23 bodies 1
extrude "Extrude6" add sketch "Sketch3" along normal blind 1.4 contours L113 A29 | L113 A29 L157 L161 | A29 L157 L161 | L114 L132 A28 L153 | L114 L132 A28 L153 | L114 L136 A26 L145 | L114 L136 A26 L145 | L114 L134 A27 L149 | L114 L134 A27 L149 bodies 1
sphere "SpherePrimitive7" add diameter 5 placed x (-1, 0, 0) y (0, -1, 0) z (0, 0, 1) at (-41.25, 77.5, 1.9) bodies 1
sphere "SpherePrimitive8" add diameter 5 placed x (-1, 0, 0) y (0, -1, 0) z (0, 0, 1) at (-63.75, 80, 1.9) bodies 1
sphere "SpherePrimitive9" add diameter 5 placed x (-1, 0, 0) y (0, -1, 0) z (0, 0, 1) at (-86.25, 80, 1.9) bodies 1
sphere "SpherePrimitive10" add diameter 5 placed x (-1, 0, 0) y (0, -1, 0) z (0, 0, 1) at (-108.75, 80, 1.9) bodies 1
extrude "Extrude7" cut sketch "Sketch3" along normal blind 1.4 contours L106 L107 L108 L109 L110 L111 L112 L113 L117 L118 L119 L120 L121 L122 L123 L124 L131 L162 L163 L164 | L113 A29 L143 L144 L162 L163 L164 | L113 A29 L144 L157 L161 L164 | L114 L117 A19 L131 L132 L133 A28 L141 L142 L153 | A29 L157 L158 L159 L160 L161 | L114 L116 A15 A19 L133 L134 L135 A27 L139 L140 L149 | L113 A29 L143 L157 L161 | A21 | L114 L115 L116 A15 L135 L136 A26 L137 L138 L145 | L114 L132 A28 L141 L142 L153 L154 L155 L156 | L114 L136 A26 L137 L138 L145 L146 L147 L148 | L114 L134 A27 L139 L140 L149 L150 L151 L152 bodies 1
extrude "Extrude8" cut sketch "Sketch3" along normal blind 1.4 contours A14 bodies 1
delete_face "DeleteFace7" 1 faces at (-42.635, 77.2128, -0.1614) on bodies 1
delete_face "DeleteFace8" 1 faces at (-65.135, 79.7128, -0.1614) on bodies 1
delete_face "DeleteFace9" 1 faces at (-87.635, 79.7128, -0.1614) on bodies 1
delete_face "DeleteFace10" 1 faces at (-110.135, 79.7128, -0.1614) on bodies 1
extrude "Extrude9" cut sketch "Sketch3" along normal blind 1.4 contours A20 bodies 1
extrude "Extrude10" add sketch "Sketch3" along normal blind 2 contours A21 bodies 1
extrude "Extrude11" cut 1 faces at (-111.3216, 67.9482, 2.5) along direction (0, 0, -1) blind 2 on bodies 1 bodies 1
extrude "Extrude12" cut 1 faces at (-91.3216, 67.9482, 1.9) along direction (0, 0, -1) blind 1.5 on bodies 1 bodies 1
extrude "Extrude13" add 1 faces at (-91.3216, 67.9482, 0.4) along direction (0, 0, 1) blind 0.1 on bodies 1 bodies 1
extrude "Extrude14" cut 1 faces at (-71.3216, 67.9482, 1.9) along direction (0, 0, -1) blind 1.4 on bodies 1 bodies 1